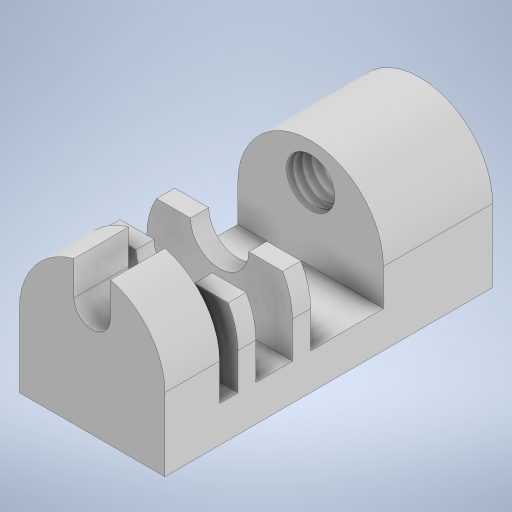
# Autodesk Inventor part: Extractor Body
Saved by Autodesk Inventor 2023 (Build 270158030, 158C)
## iProperties
Created: 2022-11-22
Part Number: Extractor Body
Material: Generic
Document SubType Name: Modeling
Designer: Imogen Heard
Density: 1 g/cm^3
Appearance: Default
Author: Imogen Heard
Autodesk Inventor part; units mm, degrees
ref_plane "YZ Plane" through (0, 0, 0) normal (1, 0, 0) x (0, 1, 0)
ref_plane "XZ Plane" through (0, 0, 0) normal (0, 1, 0) x (-1, 0, 0)
ref_plane "XY Plane" through (0, 0, 0) normal (0, 0, 1) x (1, 0, 0)
sketch "Sketch1" plane through (0, 0, 0) normal (0, 0, 1) x (1, 0, 0)
  line L0 (0, 20) -> (20, 20)
  line L1 (20, 20) -> (20, 0)
  line L2 (20, 0) -> (0, 0)
  line L3 (0, 0) -> (0, 20)
  dimension "d0" = 20
  dimension "d1" = 20
  constraints: 8 end point, 2 parallel, 1 coincident, 1 horizontal, 1 perpendicular
  measures "d0" distance between parallel lines of L1 L3
  measures "d1" distance between parallel lines of L0 L2
extrude "Extrusion1" add sketch "Sketch1" against normal blind 45
fillet "Fillet1" radius 10 2 edges at (0, 20, -22.5) (20, 20, -22.5)
sketch "Sketch2" plane through (20, 0, 0) normal (1, 0, 0) x (0, 0, -1)
  line L0 (20, 21) -> (30, 21)
  line L1 (30, 21) -> (30, 5)
  line L2 (30, 5) -> (20, 5)
  line L3 (20, 5) -> (20, 21)
  line L4 (12.5, 21) -> (17.5, 21)
  line L5 (17.5, 21) -> (17.5, 5)
  line L6 (17.5, 5) -> (12.5, 5)
  line L7 (12.5, 5) -> (12.5, 21)
  line L8 (7.5, 21) -> (10, 21)
  line L9 (10, 21) -> (10, 5)
  line L10 (10, 5) -> (7.5, 5)
  line L11 (7.5, 5) -> (7.5, 21)
  line L12 (45, 10) -> (45, 0) projected
  line L13 (0, 0) -> (45, 0) projected
  point P0 (25, 5)
  dimension "d5" = 15
  dimension "d6" = 25
  dimension "d7" = 27.5
  dimension "d8" = 32.5
  dimension "d9" = 35
  dimension "d10" = 37.5
  dimension "d11" = 5
  dimension "d12" = 21
  constraints: 24 end point, 6 parallel, 3 horizontal, 3 horizontal alignment, 3 perpendicular, 2 point on line, 1 midpoint
  measures "d5" distance between parallel lines of L12 L1
  measures "d6" distance between parallel lines of L12 L3
  measures "d7" distance between parallel lines of L12 L5
  measures "d8" distance between parallel lines of L12 L7
  measures "d9" distance between parallel lines of L12 L9
  measures "d10" distance between parallel lines of L12 L11
  measures "d11" distance from line of L13 point (25, 5)
  measures "d12" distance between parallel lines of L13 L0
extrude "Extrusion2" cut sketch "Sketch2" against normal blind 45
sketch "Sketch3" plane through (20, 0, 0) normal (1, 0, 0) x (0, 0, -1)
  line L0 (9.5, 21) -> (20.5, 21)
  line L1 (20.5, 21) -> (20.5, 15)
  line L2 (20.5, 15) -> (9.5, 15)
  line L3 (9.5, 15) -> (9.5, 21)
  line L4 (0, 0) -> (45, 0) projected
  line L5 (10, 10) -> (10, 20) projected
  line L6 (20, 20) -> (20, 10) projected
  point P0 (15, 15)
  dimension "d15" = 15
  dimension "d16" = 6
  dimension "d17" = 0.5
  dimension "d18" = 0.5
  constraints: 8 end point, 2 parallel, 1 horizontal, 1 midpoint, 1 perpendicular
  measures "d15" distance from line of L4 point (15, 15)
  measures "d16" distance between parallel lines of L2 L0
  measures "d17" distance between parallel lines of L5 L3
  measures "d18" distance between parallel lines of L6 L1
extrude "Extrusion3" cut sketch "Sketch3" against normal blind 45
sketch "Sketch4" plane through (0, 0, -45) normal (0, 0, -1) x (-1, 0, 0)
  circle A0 centre (-10, 15) radius 2
  line L0 (-20, 0) -> (0, 0) projected
  arc A1 (0, 10) -> (-20, 10) centre (-10, 10) ccw projected
  point P0 (-10, 20)
  dimension "d21" = 4
  dimension "d22" = 15
  constraints: 1 centre point, 1 point on circle, 1 vertical alignment
  measures "d21" diameter of A0
  measures "d22" distance from line of L0 A0.centre
hole "Hole1" at (10, 15, -45) direction (0, 0, 1) diameter 6.647 depth 25 thread size "M8x1.25" class "6H" standard "ISO Metric profile"
sketch "Sketch5" plane through (0, 0, 0) normal (0, 0, 1) x (1, 0, 0)
  circle A0 centre (10, 15) radius 3.3235 projected
  arc A1 (7.5, 15) -> (12.5, 15) centre (10, 15) ccw
  line L0 (7.5, 21) -> (12.5, 21)
  line L1 (12.5, 21) -> (12.5, 15)
  line L2 (7.5, 15) -> (7.5, 21)
  point P0 (0, 0)
  dimension "d31" = 5
  dimension "d32" = 2.5
  dimension "d33" = 2.5
  dimension "d34" = 6
  constraints: 6 end point, 2 point on circle, 1 centre point, 1 concentric, 1 horizontal, 1 horizontal alignment, 1 parallel, 1 perpendicular
  measures "d31" distance between parallel lines of L1 L2
  measures "d32" distance from line of L2 A0.centre
  measures "d33" radius of A1
  measures "d34" distance from line of L0 A0.centre
extrude "Extrusion4" cut sketch "Sketch5" against normal up to surface (10 mm away) contours L1 A1 L2 A0 | A0 L2 L0 L1 picked at (9.8656, 16.0996)
sketch "Sketch6" plane through (20, 5, -20) normal (0, 0, -1) x (-1, 0, 0)
  arc A0 (7.5, 10) -> (12.5, 10) centre (10, 10) ccw projected
  circle A1 centre (10, 10) radius 4
  point P0 (20, -5)
  dimension "d37" = 8
  constraints: 1 centre point, 1 concentric
  measures "d37" diameter of A1
extrude "Extrusion5" cut sketch "Sketch6" against normal up to surface (12.5 mm away)
sketch "Sketch7" plane through (0, 0, 0) normal (0, -1, 0) x (1, 0, 0)
  circle A0 centre (10, -37.5) radius 2.5
  line L0 (20, -45) -> (0, -45) projected
  point P0 (0, 0)
  point P1 (10, -45)
  dimension "d40" = 5
  dimension "d41" = 7.5
  constraints: 1 centre point, 1 midpoint, 1 vertical alignment
  measures "d40" diameter of A0
  measures "d41" distance from line of L0 A0.centre
extrude "Extrusion6" cut sketch "Sketch7" against normal blind 10
body "Solid1"
